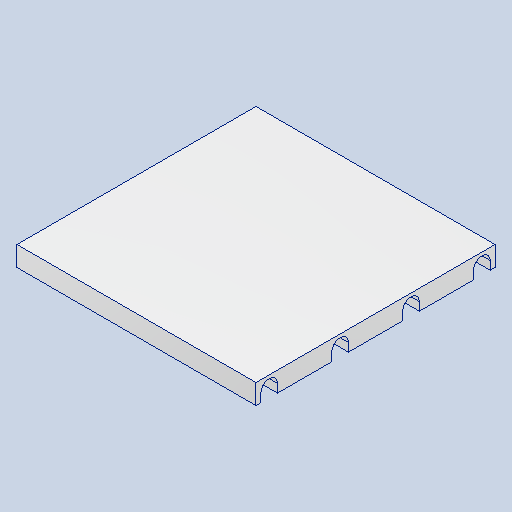
# Autodesk Inventor part: Plate
Saved by Autodesk Inventor 2022 (Build 260153000, 153)
## iProperties
Created: 2022-01-20
Part Number: Plate
Material: Aluminum 6061
Document SubType Name: Modeling
Designer: Caleb
Density: 2.7 g/cm^3
Appearance: Aluminum - Flat
Author: Caleb
Autodesk Inventor part; units mm, degrees
ref_plane "YZ Plane" through (0, 0, 0) normal (1, 0, 0) x (0, 1, 0)
ref_plane "XZ Plane" through (0, 0, 0) normal (0, 1, 0) x (-1, 0, 0)
ref_plane "XY Plane" through (0, 0, 0) normal (0, 0, 1) x (1, 0, 0)
sketch "Sketch1" plane through (0, 0, 0) normal (0, 1, 0) x (-1, 0, 0)
  line L0 (-152.4, -152.4) -> (152.4, -152.4)
  line L1 (152.4, -152.4) -> (152.4, 152.4)
  line L2 (152.4, 152.4) -> (-152.4, 152.4)
  line L3 (-152.4, 152.4) -> (-152.4, -152.4)
  line L4 (-152.4, -152.4) -> (152.4, 152.4) construction
  line L5 (152.4, -152.4) -> (-152.4, 152.4) construction
  point P0 (0, 0)
  dimension "d0" = 304.8
  dimension "d1" = 304.8
  constraints: 12 end point, 2 midpoint, 2 parallel, 1 horizontal, 1 perpendicular
  measures "d0" distance of L2.end L1.end
  measures "d1" distance of L1.end L0.end
extrude "Extrusion1" add sketch "Sketch1" along normal blind 25.4
sketch "Sketch2" plane through (152.4, 0, 152.4) normal (1, 0, 0) x (0, 0, -1)
  line L0 (304.8, 0) -> (0, 0) projected
  line L1 (6.096, 0) -> (27.432, 0)
  line L2 (27.432, 0) -> (27.432, 10.668)
  line L3 (6.096, 10.668) -> (6.096, 0)
  arc A0 (27.432, 10.668) -> (6.096, 10.668) centre (16.764, 10.668) ccw
  line L4 (0, 0) -> (0, 25.4) projected
  line L5 (117.856, 0) -> (117.856, 10.668)
  line L6 (96.52, 0) -> (117.856, 0)
  arc A1 (117.856, 10.668) -> (96.52, 10.668) centre (107.188, 10.668) ccw
  line L7 (96.52, 10.668) -> (96.52, 0)
  line L8 (208.28, 0) -> (208.28, 10.668)
  line L9 (186.944, 0) -> (208.28, 0)
  arc A2 (208.28, 10.668) -> (186.944, 10.668) centre (197.612, 10.668) ccw
  line L10 (186.944, 10.668) -> (186.944, 0)
  line L11 (298.704, 0) -> (298.704, 10.668)
  line L12 (277.368, 0) -> (298.704, 0)
  arc A3 (298.704, 10.668) -> (277.368, 10.668) centre (288.036, 10.668) ccw
  line L13 (277.368, 10.668) -> (277.368, 0)
  line L14 (304.8, 0) -> (304.8, 25.4) projected
  point P0 (152.4, 0)
  point P1 (27.432, 0)
  dimension "d4" = 10.668
  dimension "d5" = 10.668
  dimension "d6" = 6.096
  dimension "d7" = 10.668
  dimension "d10" = 90.424
  dimension "d15" = 6.096
  constraints: 24 end point, 8 point on circle, 4 centre point, 2 horizontal, 1 parallel, 1 perpendicular, 1 point on line, 1 tangent, 27 other
  measures "d4" radius of A0
  measures "d5" distance of L3.start L1.start
  measures "d6" distance between parallel lines of L4 L3
  measures "d7" distance of L1.end L2.end
  measures "d10" distance of L1.end L5.start
  measures "d15" distance between parallel lines of L14 L11
extrude "Extrusion2" cut sketch "Sketch2" against normal through all
equation "\"d7\" = d5"
body "Solid1"
